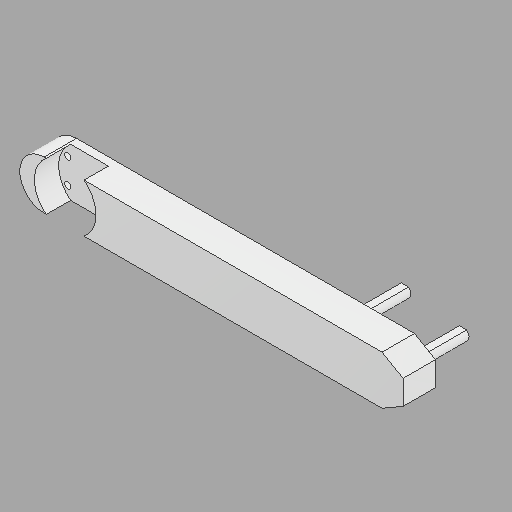
# Autodesk Inventor part: LOWER_LINKAGE
Saved by Autodesk Inventor 2025.2 (Build 292293000, 293)
## iProperties
Created: 2026-05-29
Part Number: LOWER_LINKAGE
Material: ABS Plastic
Document SubType Name: Modeling
Designer: Ben
Density: 1.06 g/cm^3
Appearance: Smooth - White
Mass: 132.026 g
Surface Area: 258.885 cm^2
Volume: 124.553 cm^3
Author: Ben
Autodesk Inventor part; units mm, degrees
ref_plane "YZ Plane" through (0, 0, 0) normal (1, 0, 0) x (0, 1, 0)
ref_plane "XZ Plane" through (0, 0, 0) normal (0, 1, 0) x (-1, 0, 0)
ref_plane "XY Plane" through (0, 0, 0) normal (0, 0, 1) x (1, 0, 0)
sketch "Sketch1" plane through (0, 0, 0) normal (0, 0, 1) x (1, 0, 0)
  circle A0 centre (0, 0) radius 15
  circle A1 centre (208.6498, 0) radius 15
  line L0 (0, 15) -> (208.6498, 15)
  line L1 (208.6498, -15) -> (0, -15)
  line L2 (208.6498, 15) -> (221.6402, 7.5)
  line L3 (221.6402, 7.5) -> (221.6402, -7.5)
  line L4 (221.6402, -7.5) -> (208.6498, -15)
  point P0 (208.6498, -15)
  dimension "d0" = 30
  dimension "d1" = 208.6498
  dimension "d16" = 180
  constraints: 10 end point, 4 point on circle, 4 tangent, 3 coincident, 2 centre point, 1 equal radius, 1 horizontal alignment, 4 other
  measures "d0" diameter of A0
  measures "d1" distance of A1.centre point (0, 0)
extrude "Extrusion1" add sketch "Sketch1" along normal blind 20 contours A0 | A0 L0 A1 L1 | L2 L3 L4 A1
sketch "Sketch2" plane through (0, 0, 0) normal (0, 0, -1) x (-1, 0, 0)
  circle A0 centre (-208.6498, 0) radius 3.75
  circle A1 centre (-167.7787, 0) radius 3.75
  line L0 (-210.8998, 3) -> (-165.5287, 3)
  line L1 (-210.8998, -3) -> (-165.5287, -3)
  line L2 (63.328, 0) -> (-274.9682, 0) projected
  line L3 (-221.6402, -7.5) -> (-221.6402, 7.5) projected
  point P0 (0, 0)
  point P1 (-170.0287, 3)
  point P2 (-170.0287, -3)
  point P3 (-206.3998, 3)
  point P4 (-206.3998, -3)
  point P5 (-208.6498, 15)
  point P6 (-221.6402, 0)
  dimension "d7" = 7.5
  dimension "d8" = 40.8711
  dimension "d11" = 6
  constraints: 4 end point, 4 point on circle, 2 centre point, 2 horizontal alignment, 1 equal radius, 1 horizontal, 1 midpoint, 1 parallel, 1 vertical alignment, 1 other
  measures "d7" diameter of A0
  measures "d8" distance of A1.centre A0.centre
  measures "d11" distance between parallel lines of L1 L0
extrude "Extrusion2" add sketch "Sketch2" along normal blind 30 contours L2 A0 L0 | A0 L1 L2 | L2 A1 L1 | A1 L0 L2
sketch "Sketch3" plane through (0, 0, 0) normal (0, 0, -1) x (-1, 0, 0)
  arc A0 (-210.8998, 3) -> (-210.8998, -3) centre (-208.6498, 0) ccw projected
  point P0 (0, 0)
  point P1 (-20, 0)
  dimension "d18" = 188.6498
  constraints: 1 horizontal alignment
  measures "d18" distance of A0.centre point (-20, 0)
hole "Hole1" at (20, 0, 0) direction (0, 0, 1) diameter 14 end through all
sketch "Sketch5" plane through (0, 0, 20) normal (0, 0, 1) x (1, 0, 0)
  circle A0 centre (20, 0) radius 7 projected
  point P0 (0, 0)
  point P1 (13, 0)
  dimension "d34" = 7
  constraints: 1 horizontal alignment
  measures "d34" distance of point (13, 0) A0.centre
hole "Hole3" at (13, 0, 20) direction (0, 0, -1) diameter 38 depth 15
sketch "Sketch6" plane through (1.3381, -15, 5) normal (0, 0, 1) x (1, 0, 0)
  arc A0 (23.3238, 0) -> (23.3238, 30) centre (11.6619, 15) ccw construction
  line L0 (30.6619, 15) -> (-7.3381, 15) construction
  arc A1 (0, 30) -> (0, 0) centre (11.6619, 15) ccw construction
  circle A2 centre (11.6619, 15) radius 15.5 construction
  point P0 (-1.3381, 15)
  point P1 (25.0853, 22.75)
  point P2 (25.0853, 7.25)
  point P3 (-1.7615, 22.75)
  point P4 (-1.7615, 7.25)
  dimension "d42" = 15.5
  dimension "d43" = 31
  dimension "d44" = 15.5
  constraints: 5 point on circle, 2 end point, 2 symmetric about line, 1 centre point, 1 coincident, 1 horizontal, 1 horizontal alignment
  measures "d42" distance of A2.start point (25.085, 22.75)
  measures "d43" diameter of A2
  measures "d44" distance of A2.end point (-1.761, 7.25)
hole "Hole4" at (26.4234, 7.75, 5) at (26.4234, -7.75, 5) at (-0.4234, 7.75, 5) at (-0.4234, -7.75, 5) direction (0, 0, -1) diameter 4 end through all
sketch "Sketch7" plane through (0, 0, -30) normal (0, 0, -1) x (-1, 0, 0)
  line L0 (-165.5287, 3) -> (-170.0287, 3) projected
  arc A0 (-170.0287, 3) -> (-170.0287, -3) centre (-167.7787, 0) ccw projected
  line L1 (-170.0287, -3) -> (-165.5287, -3) projected
  arc A1 (-165.5287, -3) -> (-165.5287, 3) centre (-167.7787, 0) ccw projected
  point P0 (0, 0)
extrude "Extrusion3" add sketch "Sketch7" along normal blind 5
body "Solid1"
